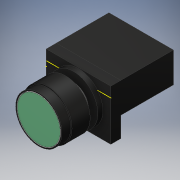
# Autodesk Inventor part: imdreset
Saved by Autodesk Inventor 2019 (Build 230136000, 136)
## iProperties
Created: 2020-02-15
Part Number: imdreset
Material: Generic
Document SubType Name: Modeling
Designer: brosemej
Density: 1 g/cm^3
Appearance: Default
Author: brosemej
Autodesk Inventor part; units mm, degrees
ref_plane "YZ Plane" through (0, 0, 0) normal (1, 0, 0) x (0, 1, 0)
ref_plane "XZ Plane" through (0, 0, 0) normal (0, 1, 0) x (-1, 0, 0)
ref_plane "XY Plane" through (0, 0, 0) normal (0, 0, 1) x (1, 0, 0)
sketch "Sketch1" plane through (0, 0, 0) normal (0, 1, 0) x (-1, 0, 0)
  line L0 (0, 0) -> (-40.64, 0)
  line L1 (-40.64, 0) -> (-40.64, -33.147)
  line L2 (-40.64, -33.147) -> (0, -33.147)
  line L3 (0, -33.147) -> (0, 0)
  dimension "d0" = 40.64
  dimension "d1" = 33.147
  constraints: 8 end point, 2 parallel, 1 horizontal, 1 perpendicular
  measures "d0" distance of L2.end L1.end
  measures "d1" distance of L1.end L0.end
extrude "Extrusion1" add sketch "Sketch1" along normal mid plane 19.05
sketch "Sketch2" plane through (0, -9.525, 0) normal (0, 0, 1) x (1, 0, 0)
  line L0 (0, -6.3625) -> (40.64, -6.3625)
  line L1 (40.64, -6.3625) -> (40.64, 12.6875)
  line L2 (40.64, 12.6875) -> (0, 12.6875)
  line L3 (0, 12.6875) -> (0, -6.3625)
  point P0 (0, 9.525)
  dimension "d4" = 40.64
  dimension "d5" = 19.05
  constraints: 8 end point, 2 parallel, 1 horizontal, 1 perpendicular
  measures "d4" distance of L2.end L1.end
  measures "d5" distance of L1.end L0.end
extrude "Extrusion2" add sketch "Sketch2" along normal blind 6.35
sketch "Sketch3" plane through (0, -9.525, 6.35) normal (0, 0, 1) x (1, 0, 0)
  line L0 (40.64, 12.6875) -> (0, 12.6875) projected
  point P0 (0, 9.525)
sketch "Sketch7" plane through (0, -9.525, 6.35) normal (0, 0, 1) x (1, 0, 0)
  point P0 (0, 9.525)
sketch "Sketch8" plane through (0, -15.8875, 0) normal (0, -1, 0) x (1, 0, 0)
  line L0 (40.64, 6.35) -> (0, 6.35) projected
  line L1 (40.64, 0) -> (0, 0) projected
  line L2 (0, 6.35) -> (40.64, 6.35)
  line L3 (40.64, 6.35) -> (40.64, 0)
  line L4 (40.64, 0) -> (0, 0)
  line L5 (0, 0) -> (0, 6.35)
  constraints: 8 end point, 2 parallel, 1 horizontal, 1 perpendicular
extrude "Extrusion5" add sketch "Sketch8" along normal blind 6.35
sketch "Sketch9" plane through (0, 3.1625, 0) normal (0, 1, 0) x (1, 0, 0)
  line L0 (40.64, 0) -> (40.64, -6.35) projected
  line L1 (0, 33.147) -> (0, 0) projected
  line L2 (40.64, -6.35) -> (0, -6.35)
  line L3 (0, -6.35) -> (0, 0)
  line L4 (0, 0) -> (40.64, 0)
  line L5 (40.64, 0) -> (40.64, -6.35)
  constraints: 8 end point, 2 parallel, 1 horizontal, 1 perpendicular
extrude "Extrusion6" add sketch "Sketch9" along normal blind 6.35
sketch "Sketch10" plane through (0, -9.525, 6.35) normal (0, 0, 1) x (1, 0, 0)
  line L0 (0, 9.525) -> (0, 19.05) projected
  circle A0 centre (20.32, 3.175) radius 15.3561
  constraints: 1 centre point
extrude "Extrusion7" add sketch "Sketch10" along normal blind 3.175
sketch "Sketch11" plane through (20.32, -6.35, 9.525) normal (0, 0, 1) x (1, 0, 0)
  circle A0 centre (0, 0) radius 9.525
  point P0 (-20.32, 6.35)
  dimension "d27" = 19.05
  constraints: 1 centre point
  measures "d27" diameter of A0
extrude "Extrusion8" add sketch "Sketch11" along normal blind 4.826
sketch "Sketch12" plane through (20.32, -6.35, 14.351) normal (0, 0, 1) x (1, 0, 0)
  circle A0 centre (0, 0) radius 15.3561
  point P0 (-20.32, 6.35)
  constraints: 1 centre point
extrude "Extrusion9" add sketch "Sketch12" along normal blind 11.43
sketch "Sketch13" plane through (20.32, -6.35, 25.781) normal (0, 0, 1) x (1, 0, 0)
  circle A0 centre (0, 0) radius 14.5863
  circle A1 centre (0, 0) radius 13.9111
  point P0 (-20.32, 6.35)
  constraints: 2 centre point, 1 coincident
extrude "Extrusion10" add sketch "Sketch13" along normal blind 5.588
sketch "Sketch14" plane through (20.32, -6.35, 25.781) normal (0, 0, 1) x (1, 0, 0)
  circle A0 centre (0, 0) radius 13.5059
  point P0 (-20.32, 6.35)
  constraints: 1 centre point
extrude "Extrusion11" add sketch "Sketch14" along normal blind 5.588
thread "Thread3" size "2-56 UNC" class "2A" standard "ANSI Unified Screw Threads" full length
body "Solid1"
